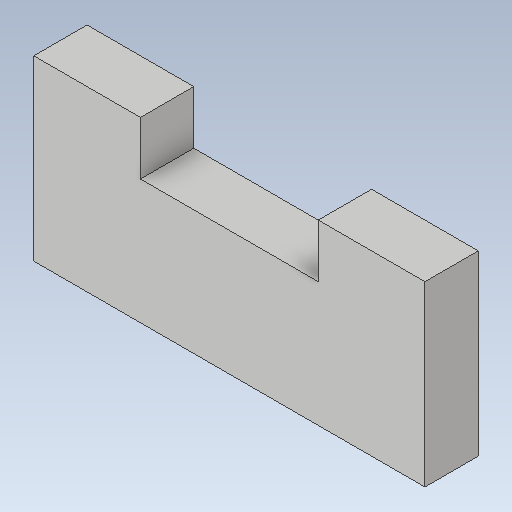
# Autodesk Inventor part: Celda sos desli
Saved by Autodesk Inventor 2020 (Build 240168000, 168)
## iProperties
Created: 2020-03-13
Part Number: Celda sos desli
Material: Genérico
Document SubType Name: Modeling
Designer: joser
Density: 1 g/cm^3
Appearance: Valor por defecto
Author: joser
Autodesk Inventor part; units mm, degrees
ref_plane "YZ Plane" through (0, 0, 0) normal (1, 0, 0) x (0, 1, 0)
ref_plane "XZ Plane" through (0, 0, 0) normal (0, 1, 0) x (-1, 0, 0)
ref_plane "XY Plane" through (0, 0, 0) normal (0, 0, 1) x (1, 0, 0)
sketch "Boceto1" plane through (0, 0, 0) normal (0, 0, 1) x (1, 0, 0)
  line L0 (22, 10) -> (22, 0)
  line L1 (22, 0) -> (0, 0)
  line L2 (0, 0) -> (0, 10)
  line L3 (6, 10) -> (6, 7)
  line L4 (6, 7) -> (16, 7)
  line L5 (16, 7) -> (16, 10)
  line L6 (0, 10) -> (6, 10)
  line L7 (16, 10) -> (22, 10)
  dimension "d0" = 22
  dimension "d1" = 10
  dimension "d3" = 10
  dimension "d4" = 6
  dimension "d5" = 3
  constraints: 16 end point, 5 perpendicular, 3 parallel, 2 horizontal, 1 coincident, 1 collinear, 1 vertical
  measures "d0" distance of L0.end L1.end
  measures "d1" distance of L0.start L0.end
  measures "d3" distance of L3.end L4.end
  measures "d4" distance between parallel lines of L2 L3
  measures "d5" distance between parallel lines of L6 L4
extrude "Extrusión1" add sketch "Boceto1" along normal blind 3
